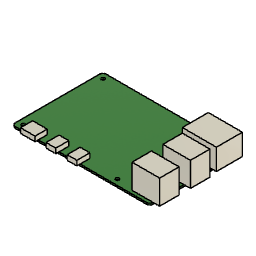
树莓派 v2 (Autodesk Fusion 360 design; units mm, degrees)
Autodesk Fusion 360 part; units mm, degrees
sketch "草图1" plane through (0, 0, 0) normal (0, 0, 1) x (1, 0, 0)
  line L0 (2, 0) -> (83, 0)
  line L1 (85, 2) -> (85, 54)
  line L2 (83, 56) -> (2, 56)
  line L3 (0, 54) -> (0, 2)
  line L4 (-9, 28) -> (96, 28)
  line L5 (32.5, 58.4958) -> (32.5, -18.5042)
  circle A0 centre (3.5, 52.5) radius 1.1
  circle A1 centre (61.5, 52.5) radius 1.1
  circle A2 centre (3.5, 3.5) radius 1.1
  circle A3 centre (61.5, 3.5) radius 1.1
  arc A4 (2, 56) -> (0, 54) centre (2, 54) ccw
  arc A5 (85, 54) -> (83, 56) centre (83, 54) ccw
  arc A6 (83, 0) -> (85, 2) centre (83, 2) ccw
  arc A7 (0, 2) -> (2, 0) centre (2, 2) ccw
  point P0 (85, 0)
  point P1 (85, 56)
  point P2 (0, 56)
  dimension "d1" = 85
  dimension "d2" = 56
  dimension "d3" = 2.2
  dimension "d4" = 49
  dimension "d5" = 58
  dimension "d6" = 3.5
  dimension "d7" = 2
  constraint horizontal L0
  constraint vertical L1
  constraint horizontal L2
  constraint vertical L3
  constraint horizontal L4
  constraint perpendicular L0 L5
  constraint symmetric L0 L2 L4
  constraint symmetric L5 A0 A1
  constraint symmetric L4 A0 A2
  constraint symmetric L4 A1 A3
  constraint coincident P2 L2
  constraint coincident P2 L3
  constraint tangent L2 A4
  constraint tangent L3 A4
  constraint coincident P1 L1
  constraint coincident P1 L2
  constraint tangent L1 A5
  constraint tangent L2 A5
  constraint equal A4 A5
  constraint coincident P0 L0
  constraint coincident P0 L1
  constraint tangent L0 A6
  constraint tangent L1 A6
  constraint equal A4 A6
  constraint tangent L0 A7
  constraint tangent L3 A7
  constraint equal A4 A7
  measures "d1" distance of P1 P2
  measures "d2" distance of P0 P1
  measures "d3" diameter of A0
  measures "d4" distance of A0.centre A2.centre
  measures "d5" distance of A0.centre A1.centre
  measures "d6" distance of L3 A2.centre
  measures "d7" radius of A4
extrude "拉伸1" add sketch "草图1" along normal blind 1 makes body 1
sketch "草图2" plane through (0, 0, 1) normal (0, 0, 1) x (-1, 0, 0)
  circle A0 centre (-3.5, -52.5) radius 1.1
  circle A1 centre (-61.5, -3.5) radius 1.1
  circle A2 centre (-61.5, -52.5) radius 1.1
  circle A3 centre (-3.5, -3.5) radius 1.1
  arc A4 (0, -2) -> (-2, 0) centre (-2, -2) ccw
  line L0 (-2, 0) -> (-83, 0)
  arc A5 (-83, 0) -> (-85, -2) centre (-83, -2) ccw
  line L1 (-85, -2) -> (-85, -54)
  arc A6 (-85, -54) -> (-83, -56) centre (-83, -54) ccw
  line L2 (-83, -56) -> (-2, -56)
  arc A7 (-2, -56) -> (0, -54) centre (-2, -54) ccw
  line L3 (0, -54) -> (0, -2)
  line L4 (-7.2, -5.5) -> (-16.2, -5.5)
  line L5 (-16.2, -5.5) -> (-16.2, 2)
  line L6 (-16.2, 2) -> (-7.2, 2)
  line L7 (-7.2, 2) -> (-7.2, -5.5)
  dimension "d10" = 3.7
  dimension "d11" = 9
  dimension "d12" = 7.5
  dimension "d13" = 5.5
  constraint horizontal L4
  constraint vertical L5
  constraint horizontal L6
  constraint vertical L7
  measures "d10" distance of A3.centre L7
  measures "d11" distance of L4.start L4.end
  measures "d12" distance of L4.end L5.end
  measures "d13" distance of L0 L4
extrude "拉伸2" add sketch "草图2" along normal blind 3 separate body contours L0 L4 L5 L7 | L0 L5 L6 L7 makes body 2
sketch "草图3" plane through (0, 0, 1) normal (0, 0, 1) x (-1, 0, 0)
  circle A0 centre (-3.5, -52.5) radius 1.1
  circle A1 centre (-61.5, -3.5) radius 1.1
  circle A2 centre (-61.5, -52.5) radius 1.1
  circle A3 centre (-3.5, -3.5) radius 1.1
  arc A4 (0, -2) -> (-2, 0) centre (-2, -2) ccw
  line L0 (-2, 0) -> (-83, 0)
  arc A5 (-83, 0) -> (-85, -2) centre (-83, -2) ccw
  line L1 (-85, -2) -> (-85, -54)
  arc A6 (-85, -54) -> (-83, -56) centre (-83, -54) ccw
  line L2 (-83, -56) -> (-2, -56)
  arc A7 (-2, -56) -> (0, -54) centre (-2, -54) ccw
  line L3 (0, -54) -> (0, -2)
  line L4 (-67, -54) -> (-88, -54)
  line L5 (-88, -54) -> (-88, -38)
  line L6 (-88, -38) -> (-67, -38)
  line L7 (-67, -38) -> (-67, -54)
  dimension "d16" = 21
  dimension "d17" = 16
  dimension "d18" = 2
  dimension "d19" = 18
  constraint horizontal L4
  constraint vertical L5
  constraint horizontal L6
  constraint vertical L7
  measures "d16" distance of L4.start L4.end
  measures "d17" distance of L4.start L6.end
  measures "d18" distance of L2 L4
  measures "d19" distance of L1 L7
extrude "拉伸3" add sketch "草图3" along normal blind 13 separate body contours L1 L4 L6 L7 | L1 L4 L5 L6 makes body 3
sketch "草图4" plane through (0, 0, 1) normal (0, 0, 1) x (-1, 0, 0)
  circle A0 centre (-3.5, -52.5) radius 1.1
  circle A1 centre (-61.5, -3.5) radius 1.1
  circle A2 centre (-61.5, -52.5) radius 1.1
  circle A3 centre (-3.5, -3.5) radius 1.1
  arc A4 (0, -2) -> (-2, 0) centre (-2, -2) ccw
  line L0 (-2, 0) -> (-83, 0)
  arc A5 (-83, 0) -> (-85, -2) centre (-83, -2) ccw
  line L1 (-85, -2) -> (-85, -54)
  arc A6 (-85, -54) -> (-83, -56) centre (-83, -54) ccw
  line L2 (-83, -56) -> (-2, -56)
  arc A7 (-2, -56) -> (0, -54) centre (-2, -54) ccw
  line L3 (0, -54) -> (0, -2)
  line L4 (-72, -33) -> (-89, -33)
  line L5 (-89, -33) -> (-89, -21)
  line L6 (-89, -21) -> (-72, -21)
  line L7 (-72, -21) -> (-72, -33)
  dimension "d22" = 17
  dimension "d23" = 12
  dimension "d24" = 13
  dimension "d25" = 21
  constraint horizontal L4
  constraint vertical L5
  constraint horizontal L6
  constraint vertical L7
  measures "d22" distance of L4.start L4.end
  measures "d23" distance of L4.start L6.end
  measures "d24" distance of L1 L7
  measures "d25" distance of L0 L6
extrude "拉伸4" add sketch "草图4" along normal blind 15 separate body contours L1 L4 L6 L7 | L1 L4 L5 L6 makes body 4
sketch "草图5" plane through (0, 0, 1) normal (0, 0, 1) x (-1, 0, 0)
  circle A0 centre (-3.5, -52.5) radius 1.1
  circle A1 centre (-61.5, -3.5) radius 1.1
  circle A2 centre (-61.5, -52.5) radius 1.1
  circle A3 centre (-3.5, -3.5) radius 1.1
  arc A4 (0, -2) -> (-2, 0) centre (-2, -2) ccw
  line L0 (-2, 0) -> (-83, 0)
  arc A5 (-83, 0) -> (-85, -2) centre (-83, -2) ccw
  line L1 (-85, -2) -> (-85, -54)
  arc A6 (-85, -54) -> (-83, -56) centre (-83, -54) ccw
  line L2 (-83, -56) -> (-2, -56)
  arc A7 (-2, -56) -> (0, -54) centre (-2, -54) ccw
  line L3 (0, -54) -> (0, -2)
  line L4 (-72, -14) -> (-89, -14)
  line L5 (-89, -14) -> (-89, -2)
  line L6 (-89, -2) -> (-72, -2)
  line L7 (-72, -2) -> (-72, -14)
  dimension "d28" = 17
  dimension "d29" = 12
  dimension "d30" = 13
  dimension "d31" = 2
  constraint horizontal L4
  constraint vertical L5
  constraint horizontal L6
  constraint vertical L7
  measures "d28" distance of L4.start L4.end
  measures "d29" distance of L4.start L6.end
  measures "d30" distance of L1 L7
  measures "d31" distance of L0 L6
extrude "拉伸5" add sketch "草图5" along normal blind 15 separate body contours L1 L4 L6 L7 | L1 L4 L5 L6 makes body 5
sketch "草图6" plane through (0, 0, 1) normal (0, 0, 1) x (-1, 0, 0)
  circle A0 centre (-3.5, -52.5) radius 1.1
  circle A1 centre (-61.5, -3.5) radius 1.1
  circle A2 centre (-61.5, -52.5) radius 1.1
  circle A3 centre (-3.5, -3.5) radius 1.1
  arc A4 (0, -2) -> (-2, 0) centre (-2, -2) ccw
  line L0 (-2, 0) -> (-83, 0)
  arc A5 (-83, 0) -> (-85, -2) centre (-83, -2) ccw
  line L1 (-85, -2) -> (-85, -54)
  arc A6 (-85, -54) -> (-83, -56) centre (-83, -54) ccw
  line L2 (-83, -56) -> (-2, -56)
  arc A7 (-2, -56) -> (0, -54) centre (-2, -54) ccw
  line L3 (0, -54) -> (0, -2)
  line L4 (-23, -6) -> (-29, -6)
  line L5 (-29, -6) -> (-29, 2)
  line L6 (-29, 2) -> (-23, 2)
  line L7 (-23, 2) -> (-23, -6)
  line L8 (-36, -6) -> (-42, -6)
  line L9 (-42, -6) -> (-42, 2)
  line L10 (-42, 2) -> (-36, 2)
  line L11 (-36, 2) -> (-36, -6)
  dimension "d34" = 8
  dimension "d35" = 8
  dimension "d36" = 6
  dimension "d37" = 6
  dimension "d38" = 6
  dimension "d39" = 6
  dimension "d40" = 23
  dimension "d41" = 36
  constraint horizontal L4
  constraint vertical L5
  constraint horizontal L6
  constraint vertical L7
  constraint horizontal L8
  constraint vertical L9
  constraint horizontal L10
  constraint vertical L11
  measures "d34" distance of L4.start L6.end
  measures "d35" distance of L8.start L10.end
  measures "d36" distance of L4.start L4.end
  measures "d37" distance of L8.start L8.end
  measures "d38" distance of L0 L4
  measures "d39" distance of L0 L8
  measures "d40" distance of L3 L7
  measures "d41" distance of L3 L11
extrude "拉伸6" add sketch "草图6" along normal blind 3 separate body contours L0 L4 L5 L7 | L0 L5 L6 L7 | L0 L8 L9 L11 | L0 L9 L10 L11 makes body 6 at (25, 3.3333, 1) makes body 7 at (38, 3.3333, 1)
copy_body "实体->零部件1" bodies 1 removing the originals makes body 8 in component "Component'"
copy_body "实体->零部件2" bodies 2 removing the originals makes body 9 in component "Component''"
copy_body "实体->零部件3" bodies 3 removing the originals makes body 10 in component "Component'''"
copy_body "实体->零部件4" bodies 4 removing the originals makes body 11 in component "Component''''"
copy_body "实体->零部件5" bodies 5 removing the originals makes body 12 in component "Component'''''"
copy_body "实体->零部件6" bodies 6 removing the originals makes body 13 in component "Component''''''"
copy_body "实体->零部件7" bodies 7 removing the originals makes body 14 in component "Component'''''''"
component "Component'" placed x (1, 0, 0) y (0, 1, 0) z (0, 0, 1) at (0, 0, 0)
component "Component''" placed x (1, 0, 0) y (0, 1, 0) z (0, 0, 1) at (0, 0, 0)
component "Component'''" placed x (1, 0, 0) y (0, 1, 0) z (0, 0, 1) at (0, 0, 0)
component "Component''''" placed x (1, 0, 0) y (0, 1, 0) z (0, 0, 1) at (0, 0, 0)
component "Component'''''" placed x (1, 0, 0) y (0, 1, 0) z (0, 0, 1) at (0, 0, 0)
component "Component''''''" placed x (1, 0, 0) y (0, 1, 0) z (0, 0, 1) at (0, 0, 0)
component "Component'''''''" placed x (1, 0, 0) y (0, 1, 0) z (0, 0, 1) at (0, 0, 0)
